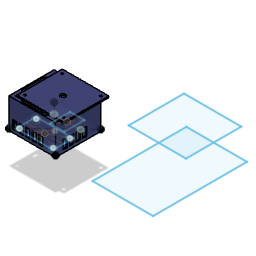
RPM Unit (Autodesk Fusion 360 design; units mm, degrees)
Autodesk Fusion 360 part; units mm, degrees
sketch "Sketch2" plane through (0, 0, 0) normal (0, 1, 0) x (1, 0, 0)
  line L0 (25, -40) -> (-40, -40)
  line L1 (-40, -40) -> (-40, 23)
  line L2 (-40, 23) -> (25, 23)
  line L3 (25, 23) -> (25, -40)
  line L4 (25, -40) -> (-40, 23) construction
  line L5 (-40, -40) -> (25, 23) construction
  dimension "d7" = 65
  dimension "d8" = 63
  constraint horizontal L0
  constraint perpendicular L0 L1
  constraint parallel L0 L2
  constraint parallel L1 L3
  measures "d7" distance of L1.end L2.end
  measures "d8" distance of L0.start L2.end
extrude "Extrude2" add sketch "Sketch2" along normal blind 2.5 makes body 1
sketch "Sketch3" plane through (0, 2.5, 0) normal (0, 1, 0) x (-1, 0, 0)
  line L0 (-25, -23) -> (40, -23)
  line L1 (40, -23) -> (40, 40)
  line L2 (40, 40) -> (-25, 40)
  line L3 (-25, 40) -> (-25, -23)
  line L4 (-16.6999, 35.0001, 0.0382) -> (35.0001, 35.0001, 0.0382)
  line L5 (35.0001, 35.0001, 0.0382) -> (35.0001, 7.0001, 0.0382)
  line L6 (35.0001, 7.0001, 0.0382) -> (-16.6999, 7.0001, 0.0382)
  line L7 (-16.6999, 7.0001, 0.0382) -> (-16.6999, 35.0001, 0.0382)
  line L8 (-16.6999, 35.0001, 0.0382) -> (35.0001, 7.0001, 0.0382) construction
  line L9 (35.0001, 35.0001, 0.0382) -> (-16.6999, 7.0001, 0.0382) construction
  circle A0 through (35.0972, 9.3001, 0.0382) (31.5016, 11.3761, 0.0382) (31.5016, 7.2242, 0.0382)
  line L10 (9.1501, 7.0001, 0.0382) -> (9.1501, 35.0001, 0.0382) construction
  line L11 (35.0001, 21.0001, 0.0382) -> (-16.6999, 21.0001, 0.0382) construction
  circle A1 through (35.0972, 32.7001, 0.0382) (31.5016, 34.7761, 0.0382) (31.5016, 30.6242, 0.0382)
  circle A2 through (-12.0028, 9.3001, 0.0382) (-15.5984, 11.3761, 0.0382) (-15.5984, 7.2242, 0.0382)
  circle A3 through (-12.0028, 32.7001, 0.0382) (-15.5984, 34.7761, 0.0382) (-15.5984, 30.6242, 0.0382)
  circle A4 through (36.5972, 9.3001, 0.0382) (30.7516, 12.6751, 0.0382) (30.7516, 5.9252, 0.0382)
  circle A5 through (36.5972, 32.7001, 0.0382) (30.7516, 36.0751, 0.0382) (30.7516, 29.3252, 0.0382)
  circle A6 through (-10.5028, 9.3001, 0.0382) (-16.3484, 12.6751, 0.0382) (-16.3484, 5.9252, 0.0382)
  circle A7 through (-10.5028, 32.7001, 0.0382) (-16.3484, 36.0751, 0.0382) (-16.3484, 29.3252, 0.0382)
  line L12 (-2.5, -22.7494) -> (-2.5, 5.2506)
  line L13 (-2.5, 5.2506) -> (17.5, 5.2506)
  line L14 (17.5, 5.2506) -> (17.5, -22.7494)
  line L15 (17.5, -22.7494) -> (-2.5, -22.7494)
  line L16 (17.5, -22.7494) -> (-2.5, 5.2506) construction
  line L17 (17.5, 5.2506) -> (-2.5, -22.7494) construction
  line L18 (26.0345, -8.7494) -> (-11.0345, -8.7494) construction
  line L19 (40, -23) -> (-25, 40) construction
  line L20 (-25, -23) -> (40, 40) construction
  line L21 (7.5, 40) -> (7.5, -23) construction
  circle A8 centre (-11.0345, -8.7494) radius 2.3971
  circle A9 centre (-11.0345, -8.7494) radius 3.8971
  circle A10 centre (26.0345, -8.7494) radius 2.3971
  circle A11 centre (26.0345, -8.7494) radius 3.8971
  point P0 (9.1501, 21.0001)
  point P1 (7.5, -8.7494)
  point P2 (7.5, 8.5)
  dimension "d18" = 51.7
  dimension "d22" = 28
  dimension "d23" = 2.3
  dimension "d24" = 2.3
  dimension "d25" = 5
  dimension "d26" = 5
  dimension "d27" = 1.5
  dimension "d223" = 4.7942
  dimension "d284" = 28
  dimension "d285" = 20
  dimension "d235" = 1.75
  dimension "d250" = 4.7942
  dimension "d253" = 1.5
  dimension "d254" = 4.7942
  dimension "d255" = 1.5
  constraint parallel L12 L14
  constraint parallel L13 L15
  constraint coincident P1 L17
  constraint coincident P1 L16
  constraint horizontal L18
  constraint coincident P1 L18
  constraint midpoint P1 L18
  constraint parallel L15 L18
  constraint vertical L14
  constraint coincident L0.end L1.start
  constraint coincident L2.end L3.start
  constraint coincident L0.start L3.end
  constraint coincident L1.end L2.start
  constraint midpoint L2 L21.start
  constraint midpoint L0 L21.end
  constraint coincident P1 L21
  constraint coincident L18.end A8.centre
  constraint concentric A8 A9
  constraint coincident L18.start A10.centre
  constraint concentric A10 A11
  measures "d284" distance of L12.start L12.end
  measures "d285" distance of L14.end L12.start
  measures "d250" diameter of A8
  measures "d253" distance of A8 A9
  measures "d254" diameter of A10
  measures "d255" distance of A10 A11
extrude "Extrude4" cut sketch "Sketch3" against normal up to surface (2.0382 mm away) from surface at -0.5 contours L4 L7 A3 A7 | L4 L7 A3 | L4 A3 | L4 L7 A3 | L7 A3 | L4 L7 A3 A7 | L4 L5 A1 A5 | L4 L5 A1 A5 | L6 L7 A2 A6 | L6 L7 A2 A6 | L4 A1 | L4 L5 A1 | L6 L7 A2 | L7 A2 | L4 L5 A1 | L5 A1 | L5 L6 A0 A4 | L5 L6 A0 A4 | L6 L7 A2 | L6 A2 | L5 A0 | L5 L6 A0 | L6 A0 | L5 L6 A0 in plane through (0, 2.5382, 0) normal (0, 1, 0) bodies 1
extrude "Extrude5" cut sketch "Sketch3" against normal up to surface (0.5 mm away) contours L4 A3 | L4 L7 A3 | L7 A3 | L4 A1 | L4 L5 A1 | L6 L7 A2 | L7 A2 | L5 A1 | L6 A2 | L5 A0 | L5 L6 A0 | L6 A0 in plane through (0, 2.5382, 0) normal (0, 1, 0) picked at (13.7675, 2.5382, 33.0253) picked at (-33.1006, 2.5382, 33.1106) picked at (15.1834, 2.5382, 9.7564) picked at (-32.514, 2.5382, 9.9216) bodies 1
extrude "Extrude6" add sketch "Sketch3" along normal blind 6.5 from surface at -0.5 contours L4 L7 A3 A7 | L4 L7 A3 | L4 L7 A3 A7 | L4 L5 A1 A5 | L4 L5 A1 A5 | L6 L7 A2 A6 | L6 L7 A2 A6 | L4 L5 A1 | L5 L6 A0 A4 | L5 L6 A0 A4 | L6 L7 A2 | L5 L6 A0 in plane through (0, 2.5382, 0) normal (0, 1, 0) picked at (16.2936, 2.5382, 34.5939) picked at (-34.5939, 2.5382, 34.5939) picked at (16.2936, 2.5382, 7.4064) picked at (-34.5939, 2.5382, 7.4064) bodies 1
chamfer "Chamfer1" distance 1 angle 45 1 edges at (-29.0668, 2.5, 10.7094) on bodies 1
chamfer "Chamfer1" distance 1 angle 45 3 edges at (-29.0668, 2.5, 34.1094) (18.0332, 2.5, 34.1094) (18.0332, 2.5, 10.7094) on bodies 1
sketch "Sketch4" plane through (0, 2.5, 0) normal (0, 1, 0) x (-1, 0, 0)
  line L0 (-23, 38) -> (38, 38)
  line L1 (38, 38) -> (38, -21)
  line L2 (38, -21) -> (-23, -21)
  line L3 (-23, -21) -> (-23, 38)
  line L4 (-23, 38) -> (38, -21) construction
  line L5 (38, 38) -> (-23, -21) construction
  line L6 (-25, -23) -> (40, -23)
  line L7 (40, 40) -> (-25, 40)
  line L8 (-25, 40) -> (-25, -23)
  line L9 (40, -23) -> (40, 40)
  line L10 (30, 8.5) -> (38, 8.5) construction
  point P0 (7.5, 8.5)
  dimension "d42" = 2
  dimension "d43" = 2
  dimension "d44" = 2
  dimension "d45" = 2
  constraint horizontal L0
  constraint perpendicular L0 L1
  constraint parallel L0 L2
  constraint parallel L1 L3
  constraint coincident L4 P0
  constraint coincident L5 P0
  constraint coincident L1 L10.end
  constraint perpendicular L1 L10
  measures "d42" distance of L1 L9
  measures "d43" distance of L3 L8
  measures "d44" distance of L2 L6
  measures "d45" distance of L0 L7
sketch "Sketch18" plane through (0, 2.5, 0) normal (0, 1, 0) x (-1, 0, 0)
  circle A0 centre (-14.3999, 32.7001) radius 4.8971
  circle A1 centre (32.7001, 9.3001) radius 4.8971
  line L0 (-25, -23) -> (40, -23)
  line L1 (40, -23) -> (40, 40)
  line L2 (40, 40) -> (-25, 40)
  line L3 (-25, 40) -> (-25, -23)
  circle A2 centre (32.7001, 32.7001) radius 4.8971
  circle A3 centre (-14.3999, 9.3001) radius 4.8971
  line L4 (32.7001, 9.3001) -> (32.7001, 10.8001) construction
  line L5 (32.7001, 10.8001) -> (28.0384, 10.8001)
  line L6 (32.7001, 10.8001) -> (28.0384, 10.8001)
  line L7 (32.7001, 32.7001) -> (32.7001, 31.2001) construction
  line L8 (32.7001, 31.2001) -> (28.0384, 31.2001)
  line L9 (32.7001, 31.2001) -> (28.0384, 31.2001)
  line L10 (32.7001, 32.7001) -> (27.8031, 32.7001)
  line L11 (32.7001, 32.7001) -> (37.5972, 32.7001)
  line L12 (32.7001, 9.3001) -> (27.8031, 9.3001)
  line L13 (32.7001, 9.3001) -> (37.5972, 9.3001)
  dimension "d140" = 1.5
  dimension "d141" = 1.5
  constraint coincident A1.centre L4.start
  constraint vertical L4
  constraint coincident A1 L5.end
  constraint perpendicular L4 L5
  constraint perpendicular L4 L6
  constraint coincident A2.centre L7.start
  constraint perpendicular L6 L7
  constraint coincident A2 L8.end
  constraint perpendicular L7 L8
  constraint perpendicular L7 L9
  constraint coincident A2 L10.end
  constraint perpendicular L7 L10
  constraint coincident A2 L11.end
  constraint perpendicular L7 L11
  constraint coincident A1 L12.end
  constraint perpendicular L4 L12
  constraint coincident A1 L13.end
  constraint perpendicular L4 L13
  measures "d140" distance of A1.centre L4.end
  measures "d141" distance of A2.centre L7.end
extrude "Extrude21" cut sketch "Sketch18" along normal up to surface (6.0382 mm away) contours A1 L12 L13 | A2 L10 L11 picked at (32.7219, 12.5557) picked at (32.7219, 29.4445) bodies 1
extrude "Extrude7" add sketch "Sketch4" along normal blind 40 from surface at -0.5 bodies 1
sketch "Sketch9" plane through (-38, 0, 0) normal (1, 0, 0) x (0, 0, -1)
  line L0 (-38, 2.5) -> (21, 2.5)
  line L1 (21, 2.5) -> (21, 42)
  line L2 (21, 42) -> (-38, 42)
  line L3 (-38, 42) -> (-38, 2.5)
  line L4 (-14.5, 3.5) -> (-27.5, 3.5)
  line L5 (-27.5, 3.5) -> (-27.5, 13.5)
  line L6 (-27.5, 13.5) -> (-14.5, 13.5)
  line L7 (-14.5, 13.5) -> (-14.5, 3.5)
  line L8 (-14.5, 3.5) -> (-27.5, 13.5) construction
  line L9 (-27.5, 3.5) -> (-14.5, 13.5) construction
  line L10 (-40, 0) -> (-40, 42)
  line L11 (-38, 2.5) -> (21, 2.5)
  point P0 (-21, 8.5)
  dimension "d71" = 19
  dimension "d72" = 6
  dimension "d73" = 10
  dimension "d74" = 13
  constraint horizontal L4
  constraint perpendicular L4 L5
  constraint parallel L4 L6
  constraint parallel L5 L7
  constraint coincident L8 P0
  constraint coincident L9 P0
  measures "d71" distance of P0 L10
  measures "d72" distance of P0 L11
  measures "d73" distance of L4 L6
  measures "d74" distance of L5.end L6.end
extrude "Extrude12" cut sketch "Sketch9" against normal up to surface (2 mm away) contours L4 L5 L6 L7 bodies 1
sketch "Sketch10" plane through (0, 42, 0) normal (0, 1, 0) x (-1, 0, 0)
  line L0 (38, -21) -> (-23, -21)
  line L1 (-23, -21) -> (-23, 38)
  line L2 (-23, 38) -> (38, 38)
  line L3 (38, 38) -> (38, -21)
  line L4 (40, -23) -> (40, 40)
  line L5 (40, 40) -> (-25, 40)
  line L6 (-25, 40) -> (-25, -23)
  line L7 (-25, -23) -> (40, -23)
  line L8 (-23, -21) -> (-15.9289, -13.9289)
  line L9 (-23, -21) -> (-22.9999, -21) construction
  line L10 (-15.9289, -13.9289) -> (-23, -6.8579)
  line L11 (-15.9289, -13.9289) -> (-35.9289, -13.9289) construction
  line L12 (-15.9289, -13.9289) -> (-8.8579, -21)
  line L13 (7.5, -21) -> (7.5, 38) construction
  line L14 (-23, 38) -> (38, -21) construction
  line L15 (38, 8.5) -> (-23, 8.5) construction
  line L16 (-15.9289, 30.9289) -> (-23, 23.8579)
  line L17 (-15.9289, 30.9289) -> (-8.8579, 38)
  line L18 (30.9289, -13.9289) -> (38, -6.8579)
  line L19 (30.9289, -13.9289) -> (23.8579, -21)
  line L20 (30.9289, 30.9289) -> (38, 23.8579)
  line L21 (30.9289, 30.9289) -> (23.8579, 38)
  circle A0 centre (-19.4645, -17.4645) radius 1.5
  circle A1 centre (-19.4645, 34.4645) radius 1.5
  circle A2 centre (34.4645, -17.4645) radius 1.5
  circle A3 centre (34.4645, 34.4645) radius 1.5
  dimension "d78" = 45
  dimension "d79" = 10
  dimension "d80" = 45
  dimension "d81" = 180
  dimension "d85" = 3
  dimension "d86" = 5
  constraint horizontal L9
  constraint coincident L0.end L1.start
  constraint horizontal L11
  constraint coincident L1 L10.end
  constraint coincident L0 L12.end
  constraint midpoint L0 L13.start
  constraint midpoint L2 L13.end
  constraint coincident L1.end L2.start
  constraint coincident L0.start L3.end
  constraint midpoint L3 L15.start
  constraint midpoint L1 L15.end
  constraint symmetric L8.end L15 L16.start
  constraint symmetric L10.end L15 L16.end
  constraint symmetric L12.end L15 L17.end
  constraint symmetric L8.end L13 L18.start
  constraint symmetric L10.end L13 L18.end
  constraint symmetric L12.end L13 L19.end
  constraint symmetric L13 L16.start L20.start
  constraint symmetric L13 L16.end L20.end
  constraint symmetric L13 L17.end L21.end
  constraint coincident L8 A0.centre
  constraint symmetric L15 A0 A1
  constraint symmetric L13 A0 A2
  constraint symmetric L13 A1 A3
  measures "d78" angle of L8 L9
  measures "d79" distance of L0.end L8.end
  measures "d80" angle of L10 L11
  measures "d81" angle of L10 L12
  measures "d85" diameter of A0
  measures "d86" distance of L0.end A0.centre
extrude "Extrude13" add sketch "Sketch10" against normal blind 5 contours L0 L3 L18 L19 | L0 L8 L12 A0 | L2 L3 L20 L21 | L1 L8 L10 A0 | L8 A0 | L8 A0 | L1 L2 L16 L17 | A1 | A2 | A3 bodies 1
extrude "Extrude14" cut sketch "Sketch10" against normal up to surface (5 mm away) contours L8 A0 | L8 A0 | A1 | A2 | A3 bodies 1
sketch "Sketch11" plane through (0, 42, 0) normal (0, 1, 0) x (-1, 0, 0)
  line L0 (33.188, -27.4745) -> (-31.812, -27.4745)
  line L1 (-31.812, -27.4745) -> (-31.812, 35.5255)
  line L2 (-31.812, 35.5255) -> (33.188, 35.5255)
  line L3 (33.188, 35.5255) -> (33.188, -27.4745)
  line L4 (0.688, -27.4745) -> (0.688, 35.5255) construction
  line L5 (-31.812, 4.0255) -> (33.188, 4.0255) construction
  line L6 (31.188, -25.4745) -> (35.188, -25.4745) construction
  line L7 (35.188, -25.4745) -> (35.188, -29.4745) construction
  line L8 (35.188, -29.4745) -> (31.188, -29.4745) construction
  line L9 (31.188, -29.4745) -> (31.188, -25.4745) construction
  line L10 (31.188, -25.4745) -> (35.188, -29.4745) construction
  line L11 (35.188, -25.4745) -> (31.188, -29.4745) construction
  line L12 (31.188, -25.4745) -> (27.6525, -21.9389) construction
  line L13 (31.188, -25.4745) -> (28, -25.4745) construction
  circle A0 centre (27.6525, -21.9389) radius 1.5
  circle A1 centre (-26.2764, -21.9389) radius 1.5
  circle A2 centre (-26.2764, 29.99) radius 1.5
  circle A3 centre (27.6525, 29.99) radius 1.5
  line L14 (33.188, -27.4745) -> (-31.812, 35.5255) construction
  line L15 (-31.812, -27.4745) -> (33.188, 35.5255) construction
  point P0 (33.188, -27.4745)
  dimension "d91" = 65
  dimension "d92" = 63
  dimension "d93" = 2
  dimension "d94" = 2
  dimension "d95" = 45
  dimension "d96" = 5
  dimension "d97" = 3
  constraint horizontal L0
  constraint vertical L1
  constraint horizontal L2
  constraint vertical L3
  constraint midpoint L0 L4.start
  constraint midpoint L2 L4.end
  constraint midpoint L1 L5.start
  constraint midpoint L3 L5.end
  constraint horizontal L6
  constraint perpendicular L6 L7
  constraint parallel L6 L8
  constraint parallel L7 L9
  constraint coincident L10 P0
  constraint coincident L11 P0
  constraint coincident P0 L0.start
  constraint horizontal L13
  constraint coincident L12.end A0.centre
  constraint symmetric L5 A0 A3
  constraint symmetric L5 A1 A2
  measures "d91" distance of P0 L0.end
  measures "d92" distance of P0 L2.end
  measures "d93" distance of L3 L9
  measures "d94" distance of L0 L6
  measures "d95" angle of L12 L13
  measures "d96" distance of L6.start L12.end
  measures "d97" diameter of A0
extrude "Extrude15" add sketch "Sketch11" along normal blind 2 separate body makes body 2
sketch "Sketch19" plane through (25, 0, 0) normal (1, 0, 0) x (0, 0, -1)
  line L0 (-40, 42) -> (-40, 0)
  line L1 (-40, 0) -> (23, 0)
  line L2 (23, 0) -> (23, 42)
  line L3 (23, 42) -> (-40, 42)
  line L4 (23, 10) -> (-40, 10) construction
  line L5 (-5.5, 16) -> (-11.5, 16)
  line L6 (-11.5, 16) -> (-11.5, 4)
  line L7 (-11.5, 4) -> (-5.5, 4)
  line L8 (-5.5, 4) -> (-5.5, 16)
  line L9 (-5.5, 16) -> (-11.5, 4) construction
  line L10 (-11.5, 16) -> (-5.5, 4) construction
  line L11 (3.5, 16) -> (-2.5, 16)
  line L12 (-2.5, 16) -> (-2.5, 4)
  line L13 (-2.5, 4) -> (3.5, 4)
  line L14 (3.5, 4) -> (3.5, 16)
  line L15 (3.5, 16) -> (-2.5, 4) construction
  line L16 (-2.5, 16) -> (3.5, 4) construction
  line L17 (0, 0) -> (-8.5, 16) construction
  line L18 (-14.5, 16.0743) -> (-20.5, 16.0743)
  line L19 (-14.5, 4.0743) -> (-14.5, 16.0743)
  line L20 (-20.5, 16.0743) -> (-14.5, 4.0743) construction
  line L21 (-20.5, 4.0743) -> (-14.5, 4.0743)
  line L22 (-14.5, 16.0743) -> (-20.5, 4.0743) construction
  line L23 (-20.5, 16.0743) -> (-20.5, 4.0743)
  line L24 (-23.5, 15.9257) -> (-29.5, 15.9257)
  line L25 (-23.5, 3.9257) -> (-23.5, 15.9257)
  line L26 (-29.5, 15.9257) -> (-23.5, 3.9257) construction
  line L27 (-29.5, 3.9257) -> (-23.5, 3.9257)
  line L28 (-23.5, 15.9257) -> (-29.5, 3.9257) construction
  line L29 (-29.5, 15.9257) -> (-29.5, 3.9257)
  point P0 (-8.5, 10)
  point P1 (0.5, 10)
  point P2 (18, 10)
  point P3 (-27, 10)
  point P4 (-17.5, 16.0743)
  point P5 (-17.5, 10.0743)
  point P6 (-26.5, 15.9257)
  point P7 (-26.5, 9.9257)
  dimension "d146" = 10
  dimension "d147" = 6
  dimension "d148" = 12
  dimension "d149" = 6
  dimension "d150" = 12
  dimension "d151" = 3
  dimension "d242" = 6
  dimension "d243" = 12
  dimension "d244" = 6
  dimension "d245" = 12
  dimension "d246" = 3
  dimension "d247" = 3
  constraint coincident L2 L4.start
  constraint coincident L0 L4.end
  constraint perpendicular L0 L4
  constraint horizontal L5
  constraint perpendicular L5 L6
  constraint parallel L5 L7
  constraint parallel L6 L8
  constraint coincident L9 P0
  constraint coincident L10 P0
  constraint midpoint L4 P0
  constraint horizontal L11
  constraint perpendicular L11 L12
  constraint parallel L11 L13
  constraint parallel L12 L14
  constraint coincident L15 P1
  constraint coincident L16 P1
  constraint coincident L4 P1
  constraint coincident L4 P2
  constraint coincident L17.start origin
  constraint midpoint L5 L17.end
  constraint coincident L4 P3
  constraint horizontal L18
  constraint perpendicular L18 L23
  constraint parallel L18 L21
  constraint parallel L19 L23
  constraint coincident P5 L22
  constraint coincident P5 L20
  constraint midpoint P4 L18
  constraint horizontal L24
  constraint perpendicular L24 L29
  constraint parallel L24 L27
  constraint parallel L25 L29
  constraint coincident P7 L28
  constraint coincident P7 L26
  constraint midpoint P6 L24
  measures "d146" distance of L1 L4
  measures "d147" distance of L6.end L7.end
  measures "d148" distance of L5.end L6.end
  measures "d149" distance of L12.end L13.end
  measures "d150" distance of L11.end L12.end
  measures "d151" distance of L8 L12
  measures "d242" distance of L21.start L19.start
  measures "d243" distance of L18.end L21.start
  measures "d244" distance of L27.start L25.start
  measures "d245" distance of L24.end L27.start
  measures "d246" distance of L6 L19
  measures "d247" distance of L23 L25
extrude "Extrude22" cut sketch "Sketch19" against normal up to surface (2 mm away) contours L5 L6 L7 L8 | L11 L12 L13 L14 | L18 L19 L21 L23 | L24 L25 L27 L29 bodies 1
sketch "Sketch20" plane through (0, 0, 40) normal (0, 0, 1) x (1, 0, 0)
  line L0 (-40, 42) -> (-40, 0)
  line L1 (-40, 0) -> (25, 0)
  line L2 (25, 0) -> (25, 42)
  line L3 (25, 42) -> (-40, 42)
  line L4 (-40, 10) -> (25, 10) construction
  line L5 (-2, 4) -> (-8, 4)
  line L6 (-8, 4) -> (-8, 16)
  line L7 (-8, 16) -> (-2, 16)
  line L8 (-2, 16) -> (-2, 4)
  line L9 (-2, 4) -> (-8, 16) construction
  line L10 (-8, 4) -> (-2, 16) construction
  line L11 (7, 4) -> (1, 4)
  line L12 (1, 4) -> (1, 16)
  line L13 (1, 16) -> (7, 16)
  line L14 (7, 16) -> (7, 4)
  line L15 (7, 4) -> (1, 16) construction
  line L16 (1, 4) -> (7, 16) construction
  line L17 (-5, 16) -> (-5, 4) construction
  line L18 (-35, 16) -> (-35, 4)
  line L19 (-29, 16) -> (-35, 16)
  line L20 (-29, 4) -> (-29, 16)
  line L21 (-35, 4) -> (-29, 4)
  line L22 (-26, 16) -> (-26, 4)
  line L23 (-26, 4) -> (-20, 4)
  line L24 (-20, 4) -> (-20, 16)
  line L25 (-20, 16) -> (-26, 16)
  line L26 (-17, 16) -> (-17, 4)
  line L27 (-11, 16) -> (-17, 16)
  line L28 (-11, 4) -> (-11, 16)
  line L29 (-17, 4) -> (-11, 4)
  point P0 (-5, 10)
  point P1 (4, 10)
  point P2 (-5, 4)
  point P3 (-5, 16)
  point P4 (-8, 4)
  point P5 (-2, 4)
  point P6 (-2, 16)
  point P7 (-5, 10)
  dimension "d163" = 10
  dimension "d164" = 6
  dimension "d165" = 12
  dimension "d166" = 6
  dimension "d167" = 12
  dimension "d170" = 3
  dimension "d175" = 5
  dimension "d219" = 6
  dimension "d220" = 3
  dimension "d221" = 3
  dimension "d222" = 6
  constraint horizontal L4
  constraint coincident L0 L4.start
  constraint coincident L2 L4.end
  constraint horizontal L5
  constraint perpendicular L5 L6
  constraint parallel L5 L7
  constraint parallel L6 L8
  constraint coincident L9 P7
  constraint coincident L10 P7
  constraint coincident L4 P7
  constraint horizontal L11
  constraint perpendicular L11 L12
  constraint parallel L11 L13
  constraint parallel L12 L14
  constraint coincident L15 P1
  constraint coincident L16 P1
  constraint coincident L4 P1
  constraint vertical L17
  constraint midpoint L7 P3
  constraint coincident L5 P2
  constraint symmetric P5 L17 P4
  constraint symmetric P4 L17 P5
  constraint symmetric L6.end L17 P6
  constraint symmetric P7 L17 P0
  constraint symmetric L11.start L17 L26.end
  constraint symmetric L11.end L17 L28.start
  constraint symmetric L12.end L17 L27.start
  constraint symmetric L13.end L17 L26.start
  constraint symmetric P3 L17 L17.start
  constraint symmetric P2 L17 L17.end
  measures "d163" distance of L1 L4
  measures "d164" distance of L6.end P6
  measures "d165" distance of P4 L6.end
  measures "d166" distance of L12.end L13.end
  measures "d167" distance of L11.end L12.end
  measures "d170" distance of L8 L12
  measures "d175" distance of L0 L18
  measures "d219" distance of L18.start L19.start
  measures "d220" distance of L20 L22
  measures "d221" distance of L24 L26
  measures "d222" distance of L22.start L24.end
extrude "Extrude23" cut sketch "Sketch20" against normal up to surface (2 mm away) contours L5 L6 L7 L8 | L11 L12 L13 L14 | L18 L19 L20 L21 | L22 L23 L24 L25 | L26 L27 L28 L29 bodies 1
extrude "Extrude27" add sketch "Sketch3" along normal blind 8 contours L12 L13 L14 L15 bodies 1
extrude "Extrude31" cut sketch "Sketch3" against normal blind 2.5 contours A8 | A9 | A10 | A11 bodies 1
extrude "Extrude32" add sketch "Sketch3" against normal blind 1 contours A9 | A11 bodies 1
sketch "Sketch25" plane through (0, 0, -23) normal (0, 0, -1) x (-1, 0, 0)
  line L0 (-25, 42) -> (-25, 0)
  line L1 (-25, 0) -> (40, 0)
  line L2 (40, 0) -> (40, 42)
  line L3 (40, 42) -> (-25, 42)
  circle A0 centre (7.5, 19) radius 3
  line L4 (-25, 42) -> (40, 0) construction
  line L5 (40, 42) -> (-25, 0) construction
  line L6 (7.5, 42) -> (7.5, 0) construction
  point P0 (7.5, 19)
  point P1 (7.5, 19)
  point P2 (7.5, 21)
  dimension "d260" = 6
  dimension "d268" = 2
  constraint coincident L0.start L3.end
  constraint coincident L1.end L2.start
  constraint coincident L2.end L3.start
  constraint coincident L0.end L1.start
  constraint coincident P1 P0
  constraint midpoint L3 L6.start
  constraint midpoint L1 L6.end
  constraint midpoint L6 P2
  constraint coincident P1 L6
  measures "d260" diameter of A0
  measures "d268" distance of P1 P2
extrude "Extrude33" cut sketch "Sketch25" against normal blind 2 contours A0 bodies 1
sketch "Sketch26" plane through (0, 44, 0) normal (0, 1, 0) x (-1, 0, 0)
  circle A0 centre (27.6525, 29.99) radius 1.5
  circle A1 centre (-26.2764, 29.99) radius 1.5
  circle A2 centre (-26.2764, -21.9389) radius 1.5
  circle A3 centre (27.6525, -21.9389) radius 1.5
  line L0 (33.188, 35.5255) -> (-31.812, 35.5255)
  line L1 (-31.812, 35.5255) -> (-31.812, -27.4745)
  line L2 (-31.812, -27.4745) -> (33.188, -27.4745)
  line L3 (33.188, -27.4745) -> (33.188, 35.5255)
  line L4 (-31.812, -27.4745) -> (33.188, 35.5255) construction
  line L5 (33.188, -27.4745) -> (-31.812, 35.5255) construction
  circle A4 centre (0.688, 4.0255) radius 3.5
  dimension "d264" = 7
  constraint coincident L1.end L2.start
  constraint coincident L0.start L3.end
  constraint coincident L2.end L3.start
  constraint coincident L0.end L1.start
  constraint midpoint L4 A4.centre
  measures "d264" diameter of A4
extrude "Extrude34" cut sketch "Sketch26" against normal blind 2 contours A4 bodies 2
sketch "Sketch27" plane through (0, 0, 0) normal (0, 1, 0) x (1, 0, 0)
  line L0 (36.5243, 0, -42.7366) -> (121.0243, 0, -42.7366)
  line L1 (121.0243, 0, -42.7366) -> (121.0243, 131, -42.7366)
  line L2 (121.0243, 131, -42.7366) -> (36.5243, 131, -42.7366)
  line L3 (36.5243, 131, -42.7366) -> (36.5243, 0, -42.7366)
  line L4 (37.2818, 49.6944) -> (117.2818, 49.6944)
  line L5 (117.2818, 49.6944) -> (117.2818, 126.8341)
  line L6 (117.2818, 126.8341) -> (37.2818, 126.8341)
  line L7 (37.2818, 126.8341) -> (37.2818, 49.6944)
  dimension "d270" = 84.5
  dimension "d271" = 131
  dimension "d272" = 80
  constraint horizontal L4
  constraint vertical L5
  constraint horizontal L6
  constraint vertical L7
  measures "d272" distance of L5.end L6.end
equation "d23 = 0.8 mm + 1.5 mm"
named bodies: "casing body", "casing lid"
